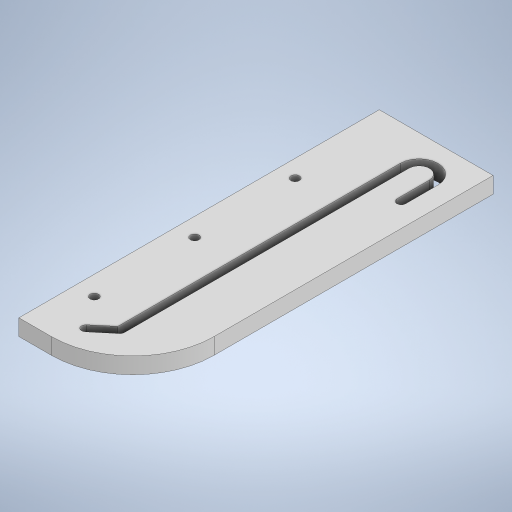
# Autodesk Inventor part: slothinge
Saved by Autodesk Inventor 2024 (Build 280153000, 153)
## iProperties
Created: 2023-09-14
Part Number: slothinge
Material: Generic
Document SubType Name: Modeling
Designer: komor
Density: 1 g/cm^3
Appearance: Default
Author: komor
Autodesk Inventor part; units mm, degrees
ref_plane "YZ Plane" through (0, 0, 0) normal (1, 0, 0) x (0, 1, 0)
ref_plane "XZ Plane" through (0, 0, 0) normal (0, 1, 0) x (-1, 0, 0)
ref_plane "XY Plane" through (0, 0, 0) normal (0, 0, 1) x (1, 0, 0)
sketch "Sketch1" plane through (0, 0, 0) normal (0, 1, 0) x (-1, 0, 0)
  line L0 (127.8549, 19.7947) -> (147.8549, 19.7947)
  line L1 (147.8549, 19.7947) -> (147.8549, 269.7947)
  line L2 (127.8549, 269.7947) -> (127.8549, 19.7947) construction
  line L3 (127.8549, 19.7947) -> (77.8549, 19.7947)
  line L4 (135.3134, 269.3194) -> (137.8549, 19.7947) construction
  circle A0 centre (136.5841, 144.5571) radius 2.65
  line L5 (136.5841, 144.5571) -> (137.8549, 19.7947) construction
  circle A1 centre (137.2195, 82.1759) radius 2.65
  line L6 (136.5841, 144.5571) -> (134.9234, 307.6106) construction
  line L7 (136.5841, 144.5571) -> (135.3134, 269.3194) construction
  circle A2 centre (135.9488, 206.9383) radius 2.65
  line L8 (110.2049, 216.8269) -> (110.2049, 41.8269) construction
  line L9 (110.2049, 216.8269) -> (121.6955, 226.4688) construction
  circle A3 centre (121.6955, 226.4688) radius 2.65
  circle A4 centre (110.2049, 216.8269) radius 2.65
  line L10 (92.3408, 41.8269) -> (92.3408, 61.8269) construction
  arc A5 (92.3408, 41.8269) -> (110.2049, 41.8269) centre (101.2728, 41.8269) ccw construction
  circle A6 centre (110.2049, 41.8269) radius 2.65
  circle A7 centre (92.3408, 61.8269) radius 2.65
  circle A8 centre (92.3408, 41.8269) radius 2.65
  line L11 (121.6955, 226.4688) -> (123.3989, 224.4387) construction
  line L12 (123.3989, 224.4387) -> (111.9082, 214.7969)
  line L13 (121.6955, 226.4688) -> (119.9921, 228.4988) construction
  line L14 (119.9921, 228.4988) -> (108.5015, 218.857)
  line L15 (110.2049, 216.8269) -> (107.5549, 216.8269) construction
  line L16 (107.5549, 216.8269) -> (107.5549, 41.8269)
  line L17 (112.8549, 41.8269) -> (112.8549, 216.8269)
  line L18 (94.9908, 61.8269) -> (94.9908, 41.8269)
  line L19 (89.6908, 61.8269) -> (89.6908, 41.8269)
  arc A9 (94.9908, 41.8269) -> (107.5549, 41.8269) centre (101.2728, 41.8269) ccw
  arc A10 (89.6908, 41.8269) -> (112.8549, 41.8269) centre (101.2728, 41.8269) ccw
  line L20 (92.3408, 61.8269) -> (94.9908, 61.8269) construction
  line L21 (77.8549, 19.7947) -> (77.8549, 191.4117)
  line L22 (112.8549, 129.3269) -> (127.8549, 129.3269) construction
  line L23 (127.8549, 241.4117) -> (147.8549, 241.4117)
  arc A11 (127.8549, 241.4117) -> (77.8549, 191.4117) centre (127.8549, 191.4117) ccw
  point P0 (0, 0)
  point P1 (112.8549, 215.5912)
  point P2 (89.6908, 41.8269)
  point P3 (77.8549, 241.4117)
  dimension "d0" = 20
  dimension "d1" = 250
  dimension "d11" = 5.3
  dimension "d12" = 5.3
  dimension "d13" = 5.3
  dimension "d16" = 175
  dimension "d17" = 15
  dimension "d18" = 130
  dimension "d19" = 5.3
  dimension "d20" = 5.3
  dimension "d21" = 20
  dimension "d22" = 5.3
  dimension "d23" = 5.3
  dimension "d24" = 5.3
  dimension "d25" = 50
  dimension "d26" = 15
  dimension "d29" = 10
  dimension "d30" = 10
  dimension "d31" = 50
  constraints: 48 end point, 21 point on circle, 13 tangent, 12 centre point, 5 coincident, 5 midpoint, 5 perpendicular, 5 point on line, 3 horizontal, 3 parallel, 3 vertical, 2 collinear
  measures "d0" distance of L2.start L1.end
  measures "d1" distance of L1.end L0.end
  measures "d11" diameter of A0
  measures "d12" diameter of A1
  measures "d13" diameter of A2
  measures "d16" distance of L8.start L8.end
  measures "d17" distance of L8.start L9.end
  measures "d18" angle of L8 L9
  measures "d19" diameter of A3
  measures "d20" diameter of A4
  measures "d21" distance of L10.start L10.end
  measures "d22" diameter of A6
  measures "d23" diameter of A7
  measures "d24" diameter of A8
  measures "d25" distance of L0.start L3.end
  measures "d26" distance of L22.start L22.end
  measures "d29" distance of L4.end L0.start
  measures "d30" distance of L0.end L4.end
  measures "d31" radius of A11
extrude "Extrusion1" add sketch "Sketch1" against normal blind 10
body "Solid1"
